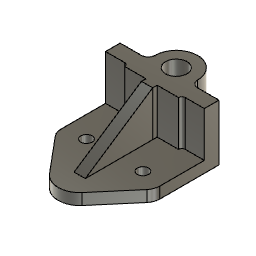
A3 v1 (Autodesk Fusion 360 design; units mm, degrees)
Autodesk Fusion 360 part; units mm, degrees
sketch "Sketch1" plane through (0, 0, 0) normal (0, 0, 1) x (1, 0, 0)
  line L0 (44, -49.5) -> (-44, -49.5)
  line L1 (-44, -49.5) -> (-44, 49.5)
  line L2 (-44, 49.5) -> (44, 49.5)
  line L3 (44, 49.5) -> (44, -49.5)
  line L4 (44, -49.5) -> (-44, 49.5) construction
  line L5 (-44, -49.5) -> (44, 49.5) construction
  line L6 (-44, 49.5) -> (-44, 36.5)
  line L7 (-44, 36.5) -> (-44, -30.5)
  circle A0 centre (-0.1186, -30.5) radius 19
  line L8 (14.358, -42.8057) -> (44, -7.9345)
  line L9 (-14.6734, -42.7129) -> (-44, -7.7628)
  line L10 (-44, -49.5) -> (-44, -7.7628)
  line L11 (44, -49.5) -> (44, -7.9345)
  circle A1 centre (-25, 0.5) radius 5
  circle A2 centre (25, 0.804) radius 5
  line L12 (-44, 49.5) -> (-44, 55.5)
  line L13 (-44, 55.5) -> (44, 55.5)
  line L14 (44, 55.5) -> (44, 49.5)
  circle A3 centre (0, 55.5) radius 9.5
  circle A4 centre (0, 55.5) radius 19
  line L15 (-18.9146, 57.2994) -> (-18.9146, 55.5)
  line L16 (-44, 36.5) -> (-24, 36.5)
  line L17 (-24, 36.5) -> (-24, 33.5)
  line L18 (-24, 33.5) -> (-5, 33.5)
  line L19 (-5, 33.5) -> (5, 33.5)
  line L20 (5, 33.5) -> (24, 33.5)
  line L21 (24, 33.5) -> (24, 36.5)
  line L22 (24, 36.5) -> (44, 36.5)
  circle A5 centre (-27, 33.5) radius 3
  circle A6 centre (27, 33.5) radius 3
  circle A7 centre (-25, 55.5) radius 6
  circle A8 centre (25, 55.5) radius 6
  line L23 (-5, 33.5) -> (-5, 29.5)
  line L24 (-5, 29.5) -> (5, 29.5)
  line L25 (5, 29.5) -> (5, 33.5)
  circle A9 centre (-31, -3.0312) radius 13
  circle A10 centre (31, -3.1558) radius 13
  dimension "d1" = 88
  dimension "d2" = 99
  dimension "d3" = 13
  dimension "d4" = 67
  dimension "d5" = 38
  dimension "d10" = 10
  dimension "d11" = 10
  dimension "d25" = 6
  dimension "d26" = 19
  dimension "d27" = 38
  dimension "d30" = 20
  dimension "d31" = 3
  dimension "d32" = 19
  dimension "d33" = 19
  dimension "d34" = 3
  dimension "d35" = 6
  dimension "d36" = 6
  dimension "d49" = 12
  dimension "d50" = 12
  dimension "d53" = 4
  dimension "d67" = 26
  dimension "d68" = 26
  constraint horizontal L0
  constraint perpendicular L0 L1
  constraint parallel L0 L2
  constraint parallel L1 L3
  constraint coincident L4 origin
  constraint coincident L5 origin
  constraint perpendicular L2 L6
  constraint parallel L1 L7
  constraint tangent L0 A0
  constraint coincident A0 L8.start
  constraint tangent A0 L8
  constraint coincident L3 L8.end
  constraint coincident A0 L9.start
  constraint coincident L7 L9.end
  constraint tangent A0 L9
  constraint perpendicular L2 L12
  constraint perpendicular L12 L13
  constraint perpendicular L13 L14
  constraint midpoint L13 A3.centre
  constraint concentric A3 A4
  constraint coincident A4 L15.start
  constraint coincident L13 L15.end
  constraint perpendicular L13 L15
  constraint perpendicular L7 L16
  constraint vertical L17
  constraint perpendicular L17 L18
  constraint parallel L18 L19
  constraint parallel L19 L20
  constraint perpendicular L20 L21
  constraint coincident L3 L22.end
  constraint perpendicular L3 L22
  constraint tangent L16 A5
  constraint tangent L17 A5
  constraint tangent L22 A6
  constraint tangent L21 A6
  constraint coincident L13 A7.centre
  constraint tangent A4 A7
  constraint coincident L13 A8.centre
  constraint tangent A4 A8
  constraint perpendicular L19 L23
  constraint perpendicular L23 L24
  constraint perpendicular L19 L25
  constraint tangent L9 A9
  constraint tangent L1 A9
  constraint tangent L8 A10
  constraint tangent L3 A10
  measures "d1" distance of L1.end L2.end
  measures "d2" distance of L0.end L1.end
  measures "d3" distance of L1.end L6.end
  measures "d4" distance of L6.end L7.end
  measures "d5" diameter of A0
  measures "d10" diameter of A1
  measures "d11" diameter of A2
  measures "d25" distance of L1.end L12.end
  measures "d26" diameter of A3
  measures "d27" diameter of A4
  measures "d30" distance of L6.end L16.end
  measures "d31" distance of L16.end L17.end
  measures "d32" distance of L17.end L18.end
  measures "d33" distance of L19.end L20.end
  measures "d34" distance of L20.end L21.end
  measures "d35" diameter of A5
  measures "d36" diameter of A6
  measures "d49" diameter of A7 L20.end
  measures "d50" diameter of A8
  measures "d53" distance of L18.end L23.end
  measures "d67" diameter of A9
  measures "d68" diameter of A10
extrude "Extrude1" add sketch "Sketch1" along normal blind 10 contours A0 | L3 L8 A10 | L1 L3 L7 A0 L8 L9 L16 L18 L20 L22 A5 A6 L23 L24 L25 A9 A10 | A10 | L1 L7 L9 A9 | A9 | L1 L2 L3 L6 A4 L16 L17 L18 L19 L20 L21 L22 | L21 L22 A6 | A6 | L16 L17 A5 | A5 | L2 A3 A4 | L19 L23 L24 L25 | L2 A3 makes body 1
fillet "Fillet1" radius 13 2 edges at (-44, -7.7628, 5) (44, -7.9345, 5) on bodies 1
extrude "Extrude2" add sketch "Sketch1" along normal blind 10 contours L2 L12 L13 A7 | L2 A4 A7 | L13 A7 picked at (-25.2846, 53.5204) bodies 1
extrude "Extrude3" cut 1 faces at (16.3818, 34.8195, 10) along direction (0, 0, -1) blind 10 on bodies 1 bodies 1
extrude "Extrude4" add sketch "Sketch1" along normal blind 10 contours A0 | L3 L8 A10 | L1 L3 L7 A0 L8 L9 L16 L18 L20 L22 A5 A6 L23 L24 L25 A9 A10 | A10 | L1 L7 L9 A9 | A9 | L19 L23 L24 L25 bodies 1
extrude "Extrude5" add sketch "Sketch1" along normal blind 10 contours A6 bodies 1
extrude "Extrude6" add sketch "Sketch1" along normal blind 10 contours A5 bodies 1
extrude "Extrude7" add sketch "Sketch1" along normal blind 50 contours L1 L2 L3 L6 A4 L16 L17 L18 L19 L20 L21 L22 | L2 L13 L14 A8 | L21 L22 A6 | L2 A4 A8 | L13 A8 | L2 L12 L13 A7 | L16 L17 A5 | L2 A4 A7 | L13 A7 picked at (25.2846, 53.5204) picked at (-25.2846, 53.5204) bodies 1
extrude "Extrude8" cut 1 faces at (-29.9293, 48.2227, 50) along direction (0, 0, -1) blind 50 on bodies 1 bodies 1
extrude "Extrude9" cut 1 faces at (4.786, -16.1011, 10) along direction (0, 0, -1) blind 10 on bodies 1 bodies 1
extrude "Extrude10" add sketch "Sketch1" along normal blind 10 contours A0 | L3 L8 A10 | L1 L3 L7 A0 L8 L9 L16 L18 L20 L22 A5 A6 L23 L24 L25 A9 A10 | A10 | L1 L7 L9 A9 | A9 | A6 | A5 bodies 1
extrude "Extrude11" add sketch "Sketch1" along normal blind 50 contours L1 L2 L3 L6 A4 L16 L17 L18 L19 L20 L21 L22 | L21 L22 A6 | L2 A4 A8 | L16 L17 A5 | L2 A3 A4 | L2 L13 A3 A4 | L13 A3 A4 L15 | L19 L23 L24 L25 | L2 A4 A7 | L2 L13 A3 A4 bodies 1
sketch "Sketch6" plane through (0, 0, 0) normal (1, 0, 0) x (0, 1, 0)
  line L0 (29.4827, 50) -> (29.4827, 10)
  line L1 (29.4827, 10) -> (-30.5173, 10)
  line L2 (-30.5173, 10) -> (29.4827, 50)
  dimension "d62" = 60
  constraint vertical L0
  constraint perpendicular L0 L1
  measures "d62" distance of L0.end L1.end
extrude "Extrude12" add sketch "Sketch6" along normal blind 5 bodies 1
extrude "Extrude13" add 1 faces at (0, 9.4827, 23.3333) along direction (-1, 0, 0) blind 5 on bodies 1 bodies 1
extrude "Extrude14" cut 1 faces at (-10, -0.1782, 10) along direction (0, 0, -1) blind 10 on bodies 1 bodies 1 makes body 2 at (9.4528, 54.5541, 16.6667)
extrude "Extrude15" cut sketch "Sketch1" along normal blind 10 contours A0 | L1 L3 L7 A0 L8 L9 L16 L18 L20 L22 A5 A6 L23 L24 L25 A9 A10 | A10 | A9 bodies 1
extrude "Extrude16" add sketch "Sketch1" along normal blind 10 contours A0 | L1 L3 L7 A0 L8 L9 L16 L18 L20 L22 A5 A6 L23 L24 L25 A9 A10 | A10 | A9 | A6 | A5 bodies 1 2
